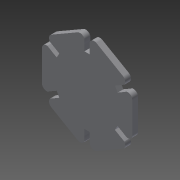
# Autodesk Inventor part: hex
Saved by Autodesk Inventor 2015 (Build 190159000, 159)
## iProperties
Created: 2015-02-16
Part Number: hex
Material: Generic
Document SubType Name: Modeling
Designer: Iain
Density: 1 g/cm^3
Appearance: Default
kerf: 0.150 mm
materialThickness: 2.500 mm
slotNoduleHeight: 0.025 mm
kercCompensation: 0.075 mm
slotWidth: 2.350 mm
slotDepth: 8.000 mm
hexWidth: 45.000 mm
Author: Iain
Autodesk Inventor part; units mm, degrees
ref_plane "YZ Plane" through (0, 0, 0) normal (1, 0, 0) x (0, 1, 0)
ref_plane "XZ Plane" through (0, 0, 0) normal (0, 1, 0) x (-1, 0, 0)
ref_plane "XY Plane" through (0, 0, 0) normal (0, 0, 1) x (1, 0, 0)
sketch "Sketch1" plane through (0, 0, 0) normal (0, 1, 0) x (-1, 0, 0)
  line L0 (19.4856, -11.25) -> (0, -22.5)
  line L1 (0, -22.5) -> (-19.4856, -11.25)
  line L2 (-19.4856, -11.25) -> (-19.4856, 11.25)
  line L3 (-19.4856, 11.25) -> (0, 22.5)
  line L4 (0, 22.5) -> (19.4856, 11.25)
  line L5 (19.4856, 11.25) -> (19.4856, -11.25)
  point P0 (0, 0)
  point P1 (0, 0)
  point P2 (19.4856, 0)
  dimension "d17" = 45
  constraints: 12 end point, 1 coincident, 1 horizontal alignment, 1 midpoint, 1 vertical alignment, 13 other
  measures "d17" distance of L3.end L0.end
extrude "Extrusion1" add sketch "Sketch1" along normal blind 2.5
sketch "Sketch2" plane through (0, 2.5, 0) normal (0, 1, 0) x (1, 0, 0)
  line L0 (-1.175, -22.5) -> (1.175, -22.5)
  line L1 (1.175, -22.5) -> (1.175, -14.5)
  line L2 (1.175, -14.5) -> (-1.175, -14.5)
  line L3 (-1.175, -14.5) -> (-1.175, -22.5)
  point P0 (0, -22.5)
  point P1 (0, 0)
  point P2 (0, -14.5)
  point P3 (0, -22.5)
  dimension "d3" = 8
  dimension "d4" = 2.35
  constraints: 8 end point, 2 midpoint, 2 parallel, 1 coincident, 1 horizontal, 1 perpendicular, 1 vertical alignment
  measures "d3" distance of L2.end L0.start
  measures "d4" distance of L1.end L2.end
extrude "Extrusion2" cut sketch "Sketch2" against normal through all
sketch "Sketch3" plane through (0, 2.5, 0) normal (0, 1, 0) x (1, 0, 0)
  line L0 (1.175, -14.5) -> (1.175, -21.8216) projected
  arc A0 (1.175, -17.1608) -> (1.175, -19.1608) centre (21.1625, -18.1608) ccw
  line L1 (1.15, -30.7617) -> (1.15, -48.4997) construction
  line L2 (1.175, -17.1608) -> (1.175, -19.1608)
  point P0 (0, 0)
  point P1 (1.175, -18.1608)
  point P2 (1.175, -18.1608)
  point P3 (1.15, -39.6307)
  point P4 (1.15, -18.1608)
  dimension "d7" = 0.025
  dimension "d8" = 1
  constraints: 4 end point, 3 midpoint, 3 point on circle, 3 vertical alignment, 1 centre point, 1 horizontal alignment, 1 parallel, 1 tangent, 1 vertical
  measures "d7" distance of point (1.175, -18.161) point (1.15, -18.161)
  measures "d8" distance of L2.start point (1.175, -18.161)
extrude "Extrusion3" add sketch "Sketch3" against normal blind 2.5
ref_plane "Work Plane1" through (0, 0, 14.5) normal (-1, 0, 0) x (0, 0, 1)
mirror "Mirror1" about plane through (0, 0, 14.5) normal (-1, 0, 0) of "Extrusion3"
sketch "Sketch4" plane through (0, 2.5, 0) normal (0, 1, 0) x (1, 0, 0)
  line L0 (1.175, -14.5) -> (1.175, -17.1608) projected
  arc A0 (1.175, -17.1608) -> (1.175, -19.1608) centre (21.1625, -18.1608) ccw projected
  line L1 (1.175, -19.1608) -> (1.175, -21.8216) projected
  line L2 (1.175, -21.8216) -> (19.4856, -11.25) projected
  line L3 (19.4856, -11.25) -> (19.4856, 11.25) projected
  line L4 (19.4856, 11.25) -> (0, 22.5) projected
  line L5 (0, 22.5) -> (-19.4856, 11.25) projected
  line L6 (-19.4856, 11.25) -> (-19.4856, -11.25) projected
  line L7 (-19.4856, -11.25) -> (-1.175, -21.8216) projected
  line L8 (-1.175, -21.8216) -> (-1.175, -19.1608) projected
  arc A1 (-1.175, -19.1608) -> (-1.175, -17.1608) centre (-21.1625, -18.1608) ccw projected
  line L9 (-1.175, -17.1608) -> (-1.175, -14.5) projected
  line L10 (-1.175, -14.5) -> (1.175, -14.5) projected
  point P0 (0, 0)
  point P1 (0, 0)
  constraints: 1 coincident
pattern_circular "Circular Pattern1" count 6 over 360 about axis through (0, 2.5, 0) along (0, 1, 0) of "Extrusion2", "Extrusion3", "Mirror1"
fillet "Fillet1" radius 2 12 edges at (-1.175, 1.25, 21.8216) (1.175, 1.25, 21.8216) (-19.4856, 1.25, 9.8932) (-18.3106, 1.25, 11.9284) (-19.4856, 1.25, -9.8932) (-18.3106, 1.25, -11.9284) (-1.175, 1.25, -21.8216) (1.175, 1.25, -21.8216) (18.3106, 1.25, -11.9284) (19.4856, 1.25, -9.8932) (19.4856, 1.25, 9.8932) (18.3106, 1.25, 11.9284)
equation "\"d17\" = hexWidth"
equation "\"d1\" = materialThickness"
equation "\"d3\" = slotDepth"
equation "\"d4\" = slotWidth"
equation "\"d5\" = materialThickness"
equation "\"d7\" = slotNoduleHeight"
equation "\"d8\" = 0.125 * slotDepth"
equation "\"d11\" = materialThickness"
equation "\"hexWidth\" = 45"
equation "\"materialThickness\" = 2.5"
equation "\"kerf\" = 0.15"
equation "\"kercCompensation\" = 0.5 * kerf"
equation "\"slotWidth\" = materialThickness - kerf"
equation "\"slotNoduleHeight\" = 0.025"
equation "\"slotDepth\" = 8"
body "Solid1"
